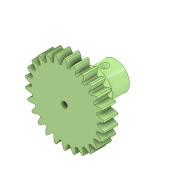
# Autodesk Inventor part: 메인 스퍼기어
Saved by Autodesk Inventor 2020 (Build 240168000, 168)
## iProperties
Created: 2020-05-04
Part Number: 메인 스퍼기어
Material: 일반
Document SubType Name: Modeling
Designer: sbahn
Density: 1 g/cm^3
Appearance: PTFE
Author: sbahn
Autodesk Inventor part; units mm, degrees
ref_plane "YZ Plane" through (0, 0, 0) normal (1, 0, 0) x (0, 1, 0)
ref_plane "XY Plane" through (0, 0, 0) normal (0, 0, 1) x (1, 0, 0)
sketch "스케치1" plane through (0, 0, 0) normal (1, 0, 0) x (0, 1, 0)
  line L0 (0, 0) -> (0, -5.8438)
  line L1 (0, 0) -> (1, 0)
  line L2 (1, 0) -> (1, -19)
  line L3 (1, -19) -> (5, -19)
  line L4 (5, -19) -> (5, -11)
  line L5 (5, -11) -> (6, -11)
  line L6 (6, -11) -> (6, -6)
  line L7 (6, -6) -> (8, -6)
  line L8 (8, -6) -> (8, 0)
  line L9 (8, 0) -> (1, 0)
  line L10 (8, -5) -> (11.75, -5)
  line L11 (11.75, -5) -> (11.75, 0)
  line L12 (11.75, 0) -> (8, 0)
  line L13 (8, 0) -> (8, -5)
  point P0 (8, 0)
  dimension "d0" = 2
  dimension "d1" = 19
  dimension "d2" = 8
  dimension "d3" = 5
  dimension "d4" = 1
  dimension "d5" = 10
  dimension "d6" = 12
  dimension "d7" = 16
  dimension "d8" = 23.5
  constraints: 28 end point, 8 perpendicular, 2 horizontal, 2 parallel, 2 vertical, 1 point on line
  measures "d0" diameter of L2 L0
  measures "d1" distance of L1.end L2.end
  measures "d2" distance of L3.end L4.end
  measures "d3" distance of L5.end L6.end
  measures "d4" distance between parallel lines of L7 L10
  measures "d5" diameter of L4 L0
  measures "d6" diameter of L6 L0
  measures "d7" diameter of L13 L0
  measures "d8" diameter of L11 L0
revolve "회전1" add sketch "스케치1" angle 360 about axis through (0, 0, 0) along (0, 0, -1)
sketch "스케치2" plane through (0, 0, 0) normal (0, 0, 1) x (1, 0, 0)
  circle A0 centre (0, 0) radius 11.75 projected
  circle A1 centre (0, 0) radius 13 construction
  circle A2 centre (0, 0) radius 14 construction
  line L0 (0, 11.75) -> (0, 14) construction
  line L1 (-0.285, 13.9971) -> (-0.285, 11.7465) construction
  line L2 (-0.785, 13.978) -> (-0.785, 11.7237) construction
  line L3 (-1.035, 13.9617) -> (-1.035, 11.7043) construction
  arc A3 (-0.285, 13.9971) -> (-1.035, 11.7043) centre (8.4443, 9.8726) ccw
  arc A4 (1.035, 11.7043) -> (0.285, 13.9971) centre (-8.4443, 9.8726) ccw
  arc A5 (0.285, 13.9971) -> (-0.285, 13.9971) centre (0, 0) ccw
  arc A6 (1.035, 11.7043) -> (-1.035, 11.7043) centre (0, 0) ccw
  point P0 (1.035, 11.7043)
  dimension "d10" = 26
  dimension "d11" = 1
  dimension "d12" = 0.5
  dimension "d13" = 0.25
  dimension "d14" = 0.785
  constraints: 17 point on circle, 8 end point, 6 centre point, 5 vertical, 3 symmetric about line, 1 coincident, 1 other
  measures "d10" diameter of A1
  measures "d11" radial gap between concentric circles of A1 A2
  measures "d12" distance between parallel lines of L2 L1
  measures "d13" distance between parallel lines of L3 L2
  measures "d14" distance between parallel lines of L0 L2
extrude "돌출1" add sketch "스케치2" against normal blind 5 contours A0 A3 A5 A4
pattern_circular "원형 패턴1" count 26 over 360 about axis through (0, 0, -2.5) along (0, 0, -1) of "돌출1"
ref_plane "작업 평면1" through (0, 5, -15) normal (0, 1, 0) x (-1, 0, 0)
sketch "스케치4" plane through (0, 5, -15) normal (0, 1, 0) x (-1, 0, 0)
  line L0 (-5, -4) -> (5, -4) projected
  line L1 (0, -4) -> (0, 1)
  point P0 (0, 15)
  dimension "d21" = 5
  constraints: 2 end point, 1 coincident, 1 midpoint, 1 vertical
  measures "d21" distance of L1.start L1.end
hole "구멍1" at (0, 5, -14) direction (0, -1, 0) diameter 3 depth 0.01 tip angle 118
sketch "스케치5" plane through (0, 0, -19) normal (0, 0, -1) x (-1, 0, 0)
  circle A0 centre (0, 0) radius 5 projected
  circle A1 centre (0, 0) radius 1 projected
extrude "돌출2" cut sketch "스케치5" against normal blind 1
